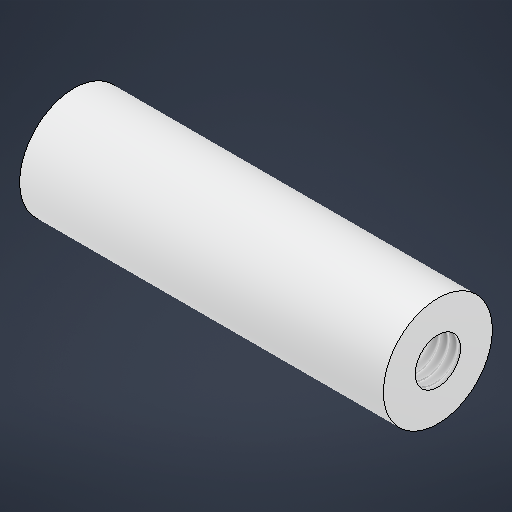
# Autodesk Inventor part: STOCK,ROUND,0.375inOD,10-32,STANDOFF
Saved by Autodesk Inventor 2026.1 (Build 301233020, 233B)
## iProperties
Created: 2026-02-16
Part Number: STOCK,ROUND,0.375inOD,10-32,STANDOFF
Material: Aluminum 6061
Document SubType Name: Modeling
Designer: Owen L
Density: 2.7 g/cm^3
Appearance: Aluminum - Flat
Author: Owen L
Autodesk Inventor part; units mm, degrees
ref_plane "YZ Plane" through (0, 0, 0) normal (1, 0, 0) x (0, 1, 0)
ref_plane "XZ Plane" through (0, 0, 0) normal (0, 1, 0) x (-1, 0, 0)
ref_plane "XY Plane" through (0, 0, 0) normal (0, 0, 1) x (1, 0, 0)
sketch "Sketch1" plane through (0, 0, 0) normal (1, 0, 0) x (0, 1, 0)
  circle A0 centre (0, 0) radius 4.7625
  dimension "d0" = 9.525
  constraints: 1 centre point, 1 coincident
  measures "d0" diameter of A0
extrude "Extrusion1" add sketch "Sketch1" along normal blind 31.8567
sketch "Sketch2" plane through (31.8567, 0, 0) normal (1, 0, 0) x (0, 0, -1)
  point P0 (0, 0)
  point P1 (0, 0)
  constraints: 1 coincident
hole "Hole1" at (31.8567, 0, 0) direction (-1, 0, 0) diameter 3.9624 depth 13.6144 tip angle 118 thread size "10-32 UNF" class "2B" standard "ANSI Unified Screw Threads"
sketch "Sketch3" plane through (0, 0, 0) normal (-1, 0, 0) x (0, 0, 1)
  circle A0 centre (0, 0) radius 1.9812 projected
  constraints: 1 coincident
hole "Hole2" at (0, 0, 0) direction (1, 0, 0) diameter 3.9624 depth 13.6144 tip angle 118 thread size "10-32 UNF" class "2B" standard "ANSI Unified Screw Threads"
body "Solid1"
